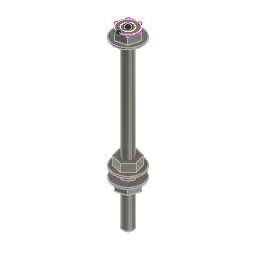
penumatic-press (Autodesk Fusion 360 archive; units mm, degrees)
design "Bolt"
Autodesk Fusion 360 part; units mm, degrees
note: some values were not read from the file. Set by a fixed rule: which face or edge a step refers to.
sketch "Sketch1" plane through (0, 0, 0) normal (0, 0, 1) x (1, 0, 0)
  line L0 (6.745515, 1.580515) -> (2.003992, 6.632045)
  line L1 (2.003992, 6.632045) -> (-4.741523, 5.05153)
  line L2 (-4.741523, 5.05153) -> (-6.745515, -1.580515)
  line L3 (-6.745515, -1.580515) -> (-2.003992, -6.632045)
  line L4 (-2.003992, -6.632045) -> (4.741523, -5.05153)
  line L5 (4.741523, -5.05153) -> (6.745515, 1.580515)
  circle A0 centre (0, 0) radius 6
  circle A1 centre (0, 0) radius 3.5
  point P0 (0, -6)
  dimension "d1" = 6
  dimension "d5" = 7
  constraint coincident A0.centre A1.centre
  constraint tangent L5 A0
  constraint coincident A0 P0
  constraint vertical A0.centre P0
  measures "d1" distance of A0.centre L5
  measures "d5" diameter of A1
extrude "Extrude1" add sketch "Sketch1" against normal blind 5 contours L0 L5 A0 | L0 L1 A0 | A0 | L4 L5 A0 | L1 L2 A0 | L3 L4 A0 | L2 L3 A0 | A1 picked at (6.169948, 1.274661) picked at (1.821767, 6.028988) picked at (4.836243, -1.779767) picked at (4.310373, -4.59219) picked at (-4.310373, 4.59219) picked at (-1.821767, -6.028988) picked at (-6.13214, -1.436797) picked at (0.901775, -0.912137) makes body 1
sketch "Sketch2" plane through (0, 0, 0) normal (1, 0, 0) x (0, 1, 0)
  line L0 (-1.580515, 0) -> (-6.632045, 0)
  line L1 (-6, 0) -> (-6.632045, 0)
  line L2 (-6.632045, 0) -> (-6.632045, -5)
  line L3 (-6.632045, 0) -> (-6.632045, -0.979962)
  arc A0 (-6, 0) -> (-6.632045, -0.979962) centre (-5.256988, -1.173025) ccw
  point P0 (-6, 0)
  point P1 (-6.632045, 0)
  constraint coincident P0 L1.start
revolve "Revolve1" cut sketch "Sketch2" angle 360 about axis through (0, 0, 1.75) along (0, 0, 1) contours L0 L1 L2 L3 A0 picked at (-6.453106, -0.226901) bodies 1
extrude "Extrude2" add sketch "Sketch1" against normal blind 110 contours A1 picked at (0.901775, -0.912137) bodies 1
thread "Thread1" "ISO Metric profile 7.0 M7x1 6g" major diameter 6.884 minor diameter 5.744 pitch 1 angle 60 resizes the face on face at (3.482608, -0.348487, -75) from (0, 0, -45) to (0, 0, -110) on bodies 1
sketch "Sketch3" plane through (0, 0, 0) normal (0, 1, 0) x (1, 0, 0)
  line L0 (3.442, 110) -> (-3.442, 110)
  line L1 (3.598063, 110) -> (3.598063, 108.649046)
  line L2 (3.598063, 108.649046) -> (1.747899, 110.436279)
  line L3 (1.747899, 110.436279) -> (3.598063, 110.436279)
  line L4 (3.598063, 110.436279) -> (3.598063, 110)
  constraint perpendicular L0 L1
  constraint perpendicular L1 L3
  constraint perpendicular L3 L4
revolve "Revolve2" cut sketch "Sketch3" angle 360 about axis through (0, 0, 1.75) along (0, 0, 1) contours L1 L2 L3 L4 picked at (3.131888, 109.549682) bodies 1
sketch "Sketch1 (2)" plane through (0, 0, 0) normal (0, 0, 1) x (1, 0, 0) in component "Nut 12mm"
  line L0 (5.997874, 3.467781) -> (-0.004249, 6.928202)
  line L1 (-0.004249, 6.928202) -> (-6.002124, 3.460421)
  line L2 (-6.002124, 3.460421) -> (-5.997874, -3.467781)
  line L3 (-5.997874, -3.467781) -> (0.004249, -6.928202)
  line L4 (0.004249, -6.928202) -> (6.002124, -3.460421)
  line L5 (6.002124, -3.460421) -> (5.997874, 3.467781)
  line L6 (4.741523, -5.05153) -> (6.745515, 1.580515)
  circle A0 centre (0, 0) radius 3.5
  dimension "d11" = 7
  constraint coincident A0.centre origin
  measures "d11" diameter of A0
extrude "Extrude1'" add sketch "Sketch1" 1 faces at (-2.496482, 0.707816, 0) along normal mid plane 5 separate body contours L0 L5 A0 | L0 L1 A0 | A0 | L4 L5 A0 | L1 L2 A0 | L3 L4 A0 | L2 L3 A0 | A1 picked at (6.169948, 1.274661) picked at (1.821767, 6.028988) picked at (4.836243, -1.779767) picked at (4.310373, -4.59219) picked at (-4.310373, 4.59219) picked at (-1.821767, -6.028988) picked at (-6.13214, -1.436797) picked at (0.901775, -0.912137) on bodies 1 makes body 2 in component "Nut 12mm"
sketch "Sketch2 (2)" plane through (0, 0, 0) normal (1, 0, 0) x (0, 1, 0) in component "Nut 12mm"
  line L0 (-6.632045, -2.5) -> (-6.632045, 2.5)
  line L1 (-1.580515, 2.5) -> (-6.632045, 2.5)
  line L2 (-6.632045, 2.5) -> (-5.871999, 2.5)
  line L3 (-6.632045, 2.5) -> (-6.632045, 1.512017)
  arc A0 (-5.871999, 2.5) -> (-6.632045, 1.512017) centre (-4.992893, 1.037373) ccw
  line L4 (-5.05153, 2.5) -> (1.580515, 2.5) construction
  line L5 (0, 0) -> (-1.735508, 2.5) construction
  dimension "d16" = 1.70649
  constraint coincident L5.start origin
  measures "d16" radius of A0
revolve "Revolve1'" cut sketch "Sketch2 (2)" angle 360 about axis through (0, 0, 1.75) along (0, 0, 1) contours L0 L1 L2 L3 A0 picked at (-6.438467, 2.216654) bodies 2 in component "Nut 12mm"
mirror "Mirror1" about plane through (0, 0, 0) normal (0, 0, 1) of "Revolve1'" in component "Nut 12mm"
extrude "Extrude2'" cut sketch "Sketch1 (2)" along normal through all and the other way through all contours A0 picked at (0.554982, -0.938125) bodies 2 in component "Nut 12mm"
thread "Thread1'" "ISO Metric profile 7.0 M7x1 6H" major diameter 7.1472 minor diameter 6.0355 pitch 1 angle 60 resizes the face on face at (3.482608, 0.348487, 1.666667) on face at (3.482608, -0.348487, -0.833333) on bodies 2 in component "Nut 12mm"
sketch "Sketch1 (3)" plane through (0, 0, 0) normal (0, 0, 1) x (1, 0, 0) in component "Washer 12mm"
  circle A0 centre (0, 0) radius 9
  circle A1 centre (0, 0) radius 4
  dimension "d18" = 18
  dimension "d19" = 8
  constraint coincident A0.centre A1.centre
  measures "d18" diameter of A0
  measures "d19" diameter of A1
extrude "Extrude1''" add sketch "Sketch1 (3)" along normal mid plane 1 separate body contours A0 picked at (7.284934, -0.64585) makes body 3 in component "Washer 12mm"
delete_face "DeleteFace1" 1 faces at (-5.028844, 3.551845, 2.285441) on bodies 2 in component "Nut 12mm"
delete_face "DeleteFace2" 1 faces at (-5.028844, 3.551845, -2.285441) on bodies 2 in component "Nut 12mm"
component "Bolt 12mm" placed x (1, 0, 0) y (0, 1, 0) z (0, 0, 1) at (0, 0, 0) in component "(Unsaved)"
component "Nut 12mm" placed x (1, 0, 0) y (0, 1, 0) z (0, 0, 1) at (0, 0, 0) in component "(Unsaved)"
component "Washer 12mm" placed x (1, 0, 0) y (0, 1, 0) z (0, 0, 1) at (0, 0, 0) in component "(Unsaved)"
component "Nut 12mm" placed x (1, 0, 0) y (0, 1, 0) z (0, 0, 1) at (0, 0, 0) in component "(Unsaved)"
component "Washer 12mm" placed x (1, 0, 0) y (0, 1, 0) z (0, 0, 1) at (0, 0, 0) in component "(Unsaved)"
component "Washer 12mm" placed x (1, 0, 0) y (0, 1, 0) z (0, 0, 1) at (0, 0, 0) in component "(Unsaved)"
